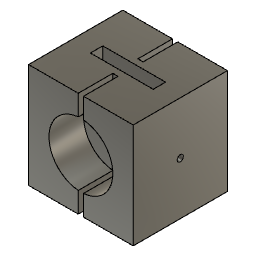
block v4 (Autodesk Fusion 360 design; units mm, degrees)
Autodesk Fusion 360 part; units mm, degrees
note: some values were not read from the file. Set by a fixed rule: which sketch regions a step uses.
sketch "Sketch1" plane through (0, 0, 0) normal (0, 0, 1) x (1, 0, 0)
  line L0 (-30.48, 114.973) -> (96.52, 114.973)
  line L1 (96.52, 114.973) -> (96.52, 0.673)
  line L2 (96.52, 0.673) -> (-30.48, 0.673)
  line L3 (-30.48, 0.673) -> (-30.48, 114.973)
  line L4 (-5.08, 65.323) -> (71.12, 65.323)
  line L5 (71.12, 65.323) -> (71.12, 50.323)
  line L6 (71.12, 50.323) -> (-5.08, 50.323)
  line L7 (-5.08, 50.323) -> (-5.08, 65.323)
  line L8 (29.845, 114.973) -> (36.195, 114.973)
  line L9 (36.195, 114.973) -> (36.195, 73.063)
  line L10 (36.195, 73.063) -> (29.845, 73.063)
  line L11 (29.845, 73.063) -> (29.845, 114.973)
  line L12 (29.845, 0.673) -> (36.195, 0.673)
  line L13 (36.195, 0.673) -> (36.195, 42.583)
  line L14 (36.195, 42.583) -> (29.845, 42.583)
  line L15 (29.845, 42.583) -> (29.845, 0.673)
  dimension "d1" = 114.3
  dimension "d2" = 127
  dimension "d3" = 15
  dimension "d4" = 76.2
  dimension "d5" = 25.4
  dimension "d8" = 49.65
  dimension "d9" = 6.35
  dimension "d10" = 60.325
  dimension "d11" = 41.91
  dimension "d12" = 41.91
  dimension "d13" = 60.325
  dimension "d14" = 6.35
  constraint horizontal L0
  constraint vertical L1
  constraint horizontal L2
  constraint vertical L3
  constraint horizontal L4
  constraint vertical L5
  constraint horizontal L6
  constraint vertical L7
  constraint horizontal L8
  constraint vertical L9
  constraint horizontal L10
  constraint vertical L11
  constraint coincident L0 L8.start
  constraint horizontal L12
  constraint vertical L13
  constraint horizontal L14
  constraint vertical L15
  constraint coincident L2 L12.start
  measures "d1" distance of L0.end L1.end
  measures "d2" distance of L0.start L0.end
  measures "d3" distance of L4.end L5.end
  measures "d4" distance of L5.end L6.end
  measures "d5" distance of L1 L5
  measures "d8" distance of L0 L4
  measures "d9" distance of L13 L15
  measures "d10" distance of L1 L13
  measures "d11" distance of L12.end L13.end
  measures "d12" distance of L8.end L9.end
  measures "d13" distance of L1 L9
  measures "d14" distance of L9.end L10.end
extrude "Extrude1" add sketch "Sketch1" along normal blind 127 contours L0 L1 L2 L3 L9 L10 L11 L13 L14 L15
sketch "Sketch2" plane through (0, 0.673, 0) normal (0, -1, 0) x (1, 0, 0)
  line L0 (-30.48, 0) -> (29.845, 0)
  line L1 (29.845, 0) -> (29.845, 127)
  line L2 (29.845, 127) -> (-30.48, 127)
  line L3 (-30.48, 127) -> (-30.48, 0)
  circle A0 centre (33.02, 63.5) radius 38.735
  dimension "d17" = 77.47
  dimension "d18" = 63.5
  dimension "d19" = 63.5
  measures "d17" diameter of A0
  measures "d18" distance of L2 A0.centre
  measures "d19" distance of L3 A0.centre
extrude "Extrude2" cut sketch "Sketch2" against normal blind 42.037 contours L1 A0 | L1 A0
sketch "Sketch3" plane through (0, 114.973, 0) normal (0, 1, 0) x (-1, 0, 0)
  line L0 (-29.845, 0) -> (30.48, 0)
  line L1 (30.48, 0) -> (30.48, 127)
  line L2 (30.48, 127) -> (-29.845, 127)
  line L3 (-29.845, 127) -> (-29.845, 0)
  circle A0 centre (-33.02, 63.5) radius 38.735
  dimension "d22" = 77.47
  dimension "d23" = 63.5
  dimension "d24" = 63.5
  measures "d22" diameter of A0
  measures "d23" distance of L1 A0.centre
  measures "d24" distance of L2 A0.centre
extrude "Extrude3" cut sketch "Sketch3" against normal blind 42.037 contours L3 A0 | L3 A0
sketch "Sketch4" plane through (96.52, 0, 0) normal (1, 0, 0) x (0, 1, 0)
  line L0 (0.673, 0) -> (114.973, 0)
  line L1 (114.973, 0) -> (114.973, 127)
  line L2 (114.973, 127) -> (0.673, 127)
  line L3 (0.673, 127) -> (0.673, 0)
  circle A0 centre (57.823, 63.5) radius 3.81
  dimension "d39" = 7.62
  dimension "d40" = 63.5
  dimension "d41" = 57.15
  measures "d39" diameter of A0
  measures "d40" distance of L2 A0.centre
  measures "d41" distance of L1 A0.centre
extrude "Extrude4" cut sketch "Sketch4" against normal blind 127 contours A0
